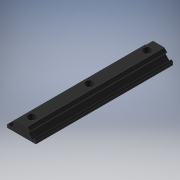
# Autodesk Inventor part: JKSGR10-95
Saved by Autodesk Inventor 2019 (Build 230136000, 136)
## iProperties
Created: 2024-06-28
Part Number: JKSGR10-95
Material: Generic
Catalog Web Link: www.cadenas.de
Description: JKSGR-Simplified Slide Guides for Jigs - Aluminum Bearing Type/Simplified Retention Type - Rail Only
Vendor: MISUMI
Document SubType Name: Modeling
Designer: psAdmin
Manufacturer: MISUMI
Mass: 8.9665 g
Surface Area: 57.72 cm^2
Volume: 8.9665 cm^3
Density: 1 g/cm^3
Appearance: PSOLRGB-175-175-175
Category: PARTsolutions
Company: MISUMI
Title: JKSGR10-95
Author: Cadenas PARTsolutions
Comments: Simplified Slide Guides for Jigs - Aluminum Bearing Type/Simplified Retention Type - Rail Only
PSOL_IDENT_0: {$CADENAS_DATA/23d-libs/misumi/metric/07_slide_rails/jksgr.prj},161 {VTYP=3D},{NB=JKSGR10-95},{LINA=
PSOL_IDENT_1: JKSGR10-95},{NN=JKSGR},{DATE=29.05.2023 01:43:56},{GEOMDATE=02.11.2021 06:14:55},{VERSION=},{LINEID=
PSOL_IDENT_2: 10},{WBVAR=L},{WBNUMERIC=L}  {NB=JKSGR10-95},{LINA=JKSGR10-95},{KT=DUMMY},{PN=JKSGR10-95},{TYPE=JKSG
PSOL_IDENT_3: R10},{MATR=Aluminum},{STR=Hard Alumite Treatment},{H=10},{L=95},{A=20},{B=30},{P1=13},{P2=13},{M=3},
PSOL_IDENT_4: {H1=7.5},{E=1.8},{DGH=3.5x6x4},{N=7.5},{P=40},{MB=F682ZZ},{SC=M2-5},{ALPB=49 (5)},{NOH=3},{L1=55,95,
PSOL_IDENT_5: 135,175,215,255,295,335,375,415,455,495,535,575,615},{D3=7.500},{D4=8.000},{DD=3.500},{G=6.000},{HH=
PSOL_IDENT_6: 4.000},{D5=3.000},{D6=2.100},{BD=4.000},{HT=10.000},{F=7.600},{D10=1.3}
NB: JKSGR10-95
NN: JKSGR
NT: Simplified Slide Guides for Jigs - Aluminum Bearing Type/Simplified Retention Type - Rail Only
NBSYN: $PN.
LINA: JKSGR10-95
CATALOG: Misumi
PN: JKSGR10-95
MATR: Aluminum
STR: Hard Alumite Treatment
H: 10
L: 95
H1: 7.5
E: 1.8
DGH: 3.5x6x4
N: 7.5
P: 40
SUPPLIER: MISUMI
ARTICLENO: JKSGR10-95
BOMINFO: JKSGR10-95
CREATOR: CADENAS GmbH
Autodesk Inventor part; units mm, degrees
sketch "_____2" plane through (0, 0, 0) normal (0, 0, 1) x (1, 0, 0)
  line L0 (-10, 1.8) -> (-10, 0)
  line L1 (-10, 0) -> (10, 0)
  line L2 (10, 0) -> (10, 1.8)
  line L3 (10, 1.8) -> (8.9929, 2.8071)
  line L4 (8.9929, 2.8071) -> (7.508, 1.3222)
  line L5 (7.508, 1.3222) -> (4.6795, 4.1506)
  line L6 (4.6795, 4.1506) -> (5.8109, 5.282)
  arc A0 (5.8109, 5.282) -> (5.8109, 5.5648) centre (5.6695, 5.4234) ccw
  line L7 (5.8109, 5.5648) -> (3.9343, 7.4414)
  arc A1 (3.9343, 7.4414) -> (3.7929, 7.5) centre (3.7929, 7.3) ccw
  line L8 (3.7929, 7.5) -> (-3.7929, 7.5)
  arc A2 (-3.7929, 7.5) -> (-3.9343, 7.4414) centre (-3.7929, 7.3) ccw
  line L9 (-3.9343, 7.4414) -> (-5.8109, 5.5648)
  arc A3 (-5.8109, 5.5648) -> (-5.8109, 5.282) centre (-5.6695, 5.4234) ccw
  line L10 (-5.8109, 5.282) -> (-4.6795, 4.1506)
  line L11 (-4.6795, 4.1506) -> (-7.508, 1.3222)
  line L12 (-7.508, 1.3222) -> (-8.9929, 2.8071)
  line L13 (-8.9929, 2.8071) -> (-10, 1.8)
  constraints: 28 end point, 8 point on circle, 4 centre point
extrude "Extrusion1" add sketch "_____2" along normal blind 95
sketch "Sketch2" plane through (-3.7929, 7.5, 0) normal (0, 1, 0) x (1, 0, 0)
  point P0 (3.7929, -7.5)
hole "Hole1" at (0, 7.5, 7.5) direction (0, -1, 0) diameter 3.5 depth 7.5 counterbore diameter 6 counterbore depth 4
pattern_linear "Rectangular Pattern1" count 3 spacing 40 along (0, 0, 1) of "Hole1"
ref_plane "to_block_XY" through (0, 0, 47.5) normal (0, 0, 1) x (1, 0, 0)
ref_plane "to_block_YZ" through (0, 0, 47.5) normal (1, 0, 0) x (0, 1, 0)
ref_plane "to_block_ZX" through (0, 0, 47.5) normal (0, 1, 0) x (0, 0, 1)
ref_plane "to_block2_XY" through (0, 0, 47.5) normal (0, 0, 1) x (1, 0, 0)
ref_plane "to_block2_YZ" through (0, 0, 47.5) normal (1, 0, 0) x (0, 1, 0)
ref_plane "to_block2_ZX" through (0, 0, 47.5) normal (0, 1, 0) x (0, 0, 1)
body "Solid1"
